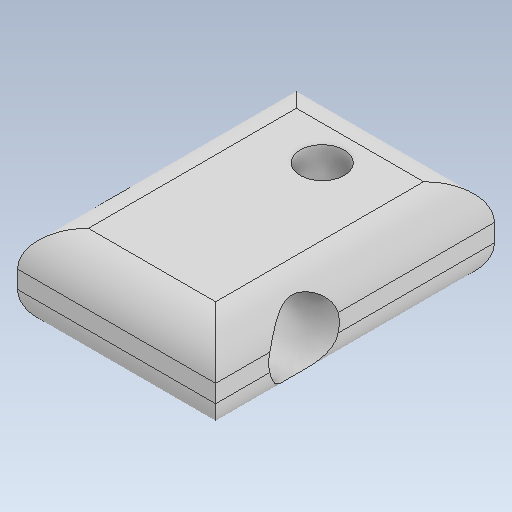
# Autodesk Inventor part: hands
Saved by Autodesk Inventor 2021 (Build 250183000, 183)
## iProperties
Created: 2021-06-27
Part Number: hands
Material: Generic
Document SubType Name: Modeling
Designer: TARUN
Density: 1 g/cm^3
Appearance: Default
Author: TARUN
Autodesk Inventor part; units mm, degrees
ref_plane "YZ Plane" through (0, 0, 0) normal (1, 0, 0) x (0, 1, 0)
ref_plane "XZ Plane" through (0, 0, 0) normal (0, 1, 0) x (-1, 0, 0)
ref_plane "XY Plane" through (0, 0, 0) normal (0, 0, 1) x (1, 0, 0)
sketch "Sketch1" plane through (0, 0, 0) normal (0, 1, 0) x (-1, 0, 0)
  line L0 (5.4006, 7.1261) -> (-5.8039, 7.1261)
  line L1 (-5.8039, 7.1261) -> (-5.8039, -8.6499)
  line L2 (-5.8039, -8.6499) -> (5.4006, -8.6499)
  line L3 (5.4006, -8.6499) -> (5.4006, 7.1261)
  point P0 (0, 0)
  constraints: 8 end point, 2 parallel, 1 horizontal, 1 perpendicular
extrude "Extrusion1" add sketch "Sketch1" along normal blind 5
sketch "Sketch2" plane through (5.8039, 0, 7.1261) normal (1, 0, 0) x (0, 0, -1)
  line L0 (0, 5) -> (15.7759, 5) projected
  circle A0 centre (5, 2.5) radius 2
  line L1 (0, 0) -> (0, 5) projected
  point P0 (7.1261, 0)
  dimension "d6" = 4
  dimension "d7" = 5
  constraints: 1 centre point
  measures "d6" diameter of A0
  measures "d7" distance from line of L1 A0.centre
extrude "Extrusion2" cut sketch "Sketch2" against normal through all
fillet "Fillet1" radius 2 8 edges at (0.2017, 5, 7.1261) (0.2017, 0, 7.1261) (-5.4006, 5, -0.7619) (0.2017, 5, -8.6499) (0.2017, 0, -8.6499) (5.8039, 0, -0.7619) (5.8039, 5, -0.7619) (-5.4006, 0, -0.7619)
sketch "Sketch3" plane through (0, 5, 0) normal (0, 1, 0) x (1, 0, 0)
  circle A0 centre (0, 4.7093) radius 1.25
  point P0 (0, 0)
  dimension "d9" = 2.5
  constraints: 1 centre point
  measures "d9" diameter of A0
extrude "Extrusion3" cut sketch "Sketch3" against normal through all
body "Solid1"
